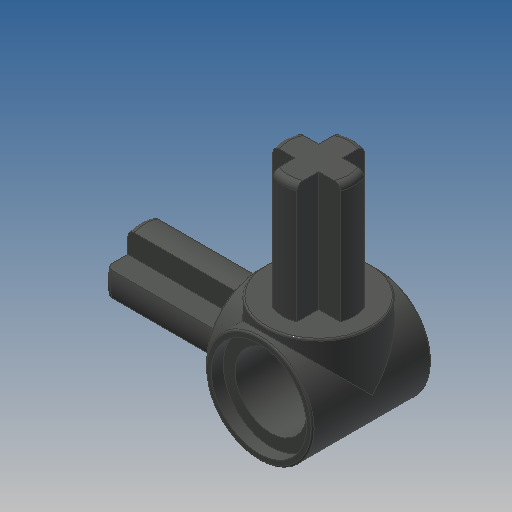
# Autodesk Inventor part: 10197-DkBluishGray
Saved by Autodesk Inventor 2022.2 (Build 262287000, 287)
## iProperties
Created: 2014-10-10
Part Number: 10197-DkBluishGray
Material: ABS Plastic
Document SubType Name: Modeling
Designer: D. Kohfeld
Mass: 0.4563 g
Surface Area: 6.87533 cm^2
Volume: 0.430472 cm^3
Density: 1.06 g/cm^3
Appearance: DkBluishGray
Author: D. Kohfeld
Autodesk Inventor part; units mm, degrees
ref_plane "YZ Plane" through (0, 0, 0) normal (1, 0, 0) x (0, 1, 0)
ref_plane "XY Plane" through (0, 0, 0) normal (0, 0, 1) x (1, 0, 0)
sketch "Sketch1" plane through (0, 0, 0) normal (0, 0, 1) x (1, 0, 0)
  circle A0 centre (0, 0) radius 3.6
  circle A1 centre (0, 0) radius 2.4
  dimension "d0" = 4.8
  dimension "d1" = 7.2
  constraints: 2 centre point, 2 coincident
  measures "d0" diameter of A1
  measures "d1" diameter of A0
extrude "Extrusion1" add sketch "Sketch1" along normal mid plane 8
sketch "Sketch4" plane through (0, 0, 4) normal (0, 0, 1) x (1, 0, 0)
  circle A0 centre (0, 0) radius 2.4 projected
  circle A1 centre (0, 0) radius 3.6 projected
  circle A2 centre (0, 0) radius 3.2
  dimension "d18" = 6.4
  constraints: 1 centre point, 1 coincident
  measures "d18" diameter of A2
extrude "Extrusion4" cut sketch "Sketch4" against normal blind 0.8 contours A2
mirror "Mirror1" about plane through (0, 0, 0) normal (0, 0, 1) of "Extrusion4"
ref_plane "Work Plane2" through (0, 4, 0) normal (0, 1, 0) x (-1, 0, 0)
sketch "Sketch2" plane through (0, 4, 0) normal (0, 1, 0) x (-1, 0, 0)
  circle A0 centre (0, 0) radius 3.6
  line L0 (-3.6, -4) -> (-3.6, 4) construction
  constraints: 1 centre point, 1 coincident, 1 tangent
extrude "Extrusion2" add sketch "Sketch2" against normal up to next
sketch "Sketch3" plane through (0, 4, 0) normal (0, 1, 0) x (1, 0, 0)
  circle A0 centre (0, 0) radius 2.4 construction
  line L0 (-0.8, 2.2627) -> (-0.8, 0.8)
  line L1 (-0.8, 0.8) -> (-2.2627, 0.8)
  line L2 (-2.2627, -0.8) -> (-0.8, -0.8)
  line L3 (-0.8, -0.8) -> (-0.8, -2.2627)
  line L4 (0.8, -2.2627) -> (0.8, -0.8)
  line L5 (0.8, -0.8) -> (2.2627, -0.8)
  line L6 (2.2627, 0.8) -> (0.8, 0.8)
  line L7 (0.8, 0.8) -> (0.8, 2.2627)
  arc A1 (0.8, 2.2627) -> (-0.8, 2.2627) centre (0, 0) ccw
  arc A2 (-2.2627, 0.8) -> (-2.2627, -0.8) centre (0, 0) ccw
  arc A3 (-0.8, -2.2627) -> (0.8, -2.2627) centre (0, 0) ccw
  arc A4 (2.2627, -0.8) -> (2.2627, 0.8) centre (0, 0) ccw
  circle A5 centre (0, 0) radius 3.6 projected
  dimension "d10" = 4.8
  dimension "d9" = 1.6
  constraints: 16 end point, 8 point on circle, 7 equal length, 4 centre point, 4 perpendicular, 3 parallel, 2 coincident, 1 vertical, 14 other
  measures "d9" distance between parallel lines of L7 L0
extrude "Extrusion3" add sketch "Sketch3" along normal blind 8 contours A1 L7 L6 A4 L5 L4 A3 L3 L2 A2 L1 L0
pattern_circular "Circular Pattern1" count 2 over 90 about axis through (0, 0, 0) along (0, 0, 1) of "Extrusion2", "Extrusion3"
fillet "Fillet1" radius 0.1 4 edges at (3.6, 4, 0) (-4, 3.6, 0) (-3.6, 0, 4) (-3.6, 0, -4)
fillet "Fillet1" radius 0.4 8 edges at (-12, 2.4, 0) (-12, 0, 2.4) (0, 12, 2.4) (-2.4, 12, 0) (0, 12, -2.4) (2.4, 12, 0) (-12, 0, -2.4) (-12, -2.4, 0)
equation "\"d0\" = tpd"
equation "\"d1\" = tlad"
equation "\"d3\" = lu"
equation "\"d18\" = tsd"
equation "\"d19\" = tsl"
equation "\"d7\" = lu"
equation "\"d10\" = kd"
equation "\"d9\" = axlet"
equation "\"d11\" = lu"
equation "\"d16\" = lf"
equation "\"d17\" = tf"
equation "\"d6\" = 0.5 * lu"
equation "\"lf\" = 0.1"
equation "\"tf\" = 0.4"
equation "\"tpd\" = 4.8"
equation "\"tlad\" = 7.2"
equation "\"lu\" = 8"
equation "\"tsd\" = 6.4"
equation "\"tsl\" = 0.8"
equation "\"kd\" = 4.8"
equation "\"axlet\" = 1.6"
body "Solid1"
